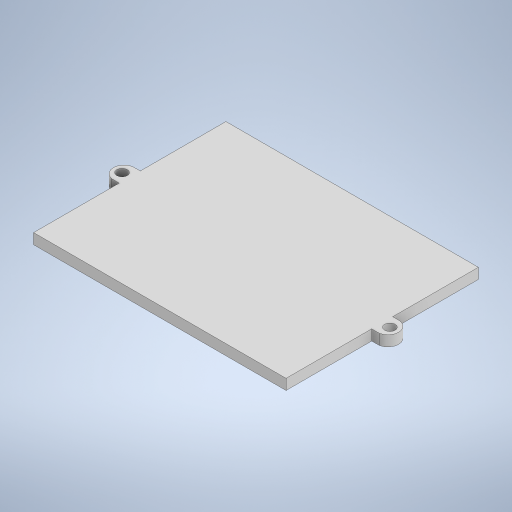
# Autodesk Inventor part: tampa_pilha
Saved by Autodesk Inventor 2024.3 (Build 283343000, 343)
## iProperties
Created: 2024-11-19
Part Number: tampa_pilha
Material: Genérico
Document SubType Name: Modeling
Designer: lostv
Density: 1 g/cm^3
Appearance: Padrão
Author: lostv
Autodesk Inventor part; units mm, degrees
ref_plane "YZ Plane" through (0, 0, 0) normal (1, 0, 0) x (0, 1, 0)
ref_plane "XZ Plane" through (0, 0, 0) normal (0, 1, 0) x (-1, 0, 0)
ref_plane "XY Plane" through (0, 0, 0) normal (0, 0, 1) x (1, 0, 0)
sketch "Esboço1" plane through (0, 0, 0) normal (0, 1, 0) x (-1, 0, 0)
  line L0 (35.5878, 45.6911) -> (-44.4122, 45.6911)
  line L1 (-44.4122, 45.6911) -> (-44.4122, -14.3089)
  line L2 (-44.4122, -14.3089) -> (35.5878, -14.3089)
  line L3 (35.5878, -14.3089) -> (35.5878, 45.6911)
  line L4 (35.5878, 45.6911) -> (35.5878, -14.3089)
  line L5 (45.5878, 15.6911) -> (-44.4122, 15.6911)
  line L6 (-4.4122, 85.6911) -> (-4.4122, -84.3089)
  line L7 (-44.4122, -14.3089) -> (-44.4122, 45.6911)
  line L8 (37.5878, 47.6911) -> (-46.4122, 47.6911)
  line L9 (-46.4122, -16.3089) -> (37.5878, -16.3089)
  circle A0 centre (40.1473, 15.6911) radius 1.75
  line L10 (40.1473, 19.1911) -> (37.5878, 19.1911)
  line L11 (37.5878, 12.1911) -> (40.1473, 12.1911)
  arc A1 (40.1473, 12.1911) -> (40.1473, 19.1911) centre (39.4884, 15.6911) ccw
  line L12 (37.5878, -16.3089) -> (37.5878, 12.1911)
  line L13 (37.5878, 19.1911) -> (37.5878, 47.6911)
  line L14 (-48.9716, 19.1911) -> (-46.4122, 19.1911)
  line L15 (-46.4122, 12.1911) -> (-48.9716, 12.1911)
  circle A2 centre (-48.9716, 15.6911) radius 1.75
  arc A3 (-48.9716, 19.1911) -> (-48.9716, 12.1911) centre (-48.3127, 15.6911) ccw
  line L16 (-46.4122, 47.6911) -> (-46.4122, 19.1911)
  line L17 (-46.4122, 12.1911) -> (-46.4122, -16.3089)
  point P0 (0, 0)
  point P1 (0.5878, 15.6911)
  point P2 (-4.4122, -16.3089)
  dimension "d2" = 60
  dimension "d3" = 30
  dimension "d4" = 80
  dimension "d5" = 64
  dimension "d6" = 32
  dimension "d7" = 3.5
  dimension "d8" = 3.5
  constraints: 36 end point, 9 parallel, 6 symmetric about line, 4 centre point, 4 perpendicular, 4 point on circle, 3 horizontal, 3 midpoint, 1 collinear, 1 point on line, 2 other
  measures "d2" distance of L3.start L3.end
  measures "d3" distance between parallel lines of L0 L5
  measures "d4" distance between parallel lines of L1 L4
  measures "d5" distance between parallel lines of L9 L8
  measures "d6" distance from line of point (0.588, 15.691) L8
  measures "d7" distance from line of A0.centre L10
  measures "d8" distance from line of A0.centre L11
extrude "Extrusão1" add sketch "Esboço1" along normal blind 3.5 contours L3 L5 L6 L0 | L0 L6 L8 L13 L10 A1 L5 A0 L3 | L6 L5 L1 L0 | L0 L1 L2 L6 L9 L17 L15 A3 L14 L16 L8 | L5 A0 A1 L11 L12 L9 L6 L2 L3 | L3 L2 L6 L5 | L6 L2 L1 L5
